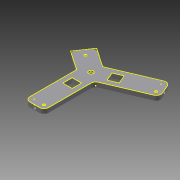
# Autodesk Inventor part: Auto Steering Part
Saved by Autodesk Inventor 2014 (Build 180170000, 170)
## iProperties
Created: 2015-01-15
Part Number: Auto Steering Part
Material: Generic
Document SubType Name: Modeling
Designer: WillHuie
Density: 1 g/cm^3
Appearance: Default
Author: WillHuie
Autodesk Inventor part; units mm, degrees
ref_plane "YZ Plane" through (0, 0, 0) normal (1, 0, 0) x (0, 1, 0)
ref_plane "XZ Plane" through (0, 0, 0) normal (0, 1, 0) x (-1, 0, 0)
ref_plane "XY Plane" through (0, 0, 0) normal (0, 0, 1) x (1, 0, 0)
sketch "Sketch1" plane through (0, 0, 0) normal (0, 1, 0) x (-1, 0, 0)
  line L0 (0, -74.6125) -> (0, -76.2)
  line L1 (0, -76.2) -> (-1.461, -76.8211)
  line L2 (-70.1269, -106.0104) -> (-75.0953, -94.3226)
  line L3 (0, 0) -> (-12.7, 0)
  line L4 (0, 0) -> (12.7, 0)
  line L5 (-75.0953, -94.3226) -> (-12.7, -67.7988)
  line L6 (-12.7, 0) -> (-12.7, -67.7988)
  line L7 (-70.1269, -106.0104) -> (-65.1585, -117.6982)
  line L8 (-65.1585, -117.6982) -> (12.7, -84.6012)
  line L9 (12.7, -84.6012) -> (12.7, 0)
  circle A0 centre (0, -76.2) radius 1.5875
  dimension "d0" = 76.2
  dimension "d1" = 76.2
  dimension "d2" = 113.03
  dimension "d3" = 12.7
  dimension "d4" = 12.7
  dimension "d5" = 12.7
  dimension "d6" = 12.7
  dimension "d7" = 3.175
  constraints: 20 end point, 6 perpendicular, 2 coincident, 2 point on circle, 1 centre point, 1 collinear, 1 parallel, 1 vertical
  measures "d0" distance of L3.start L0.end
  measures "d1" distance of L0.end L2.start
  measures "d2" angle of L0 L1
  measures "d3" distance of L2.start L2.end
  measures "d4" distance of L3.start L3.end
  measures "d5" distance of L3.start L4.end
  measures "d6" distance of L2.start L7.end
  measures "d7" diameter of A0
extrude "Extrusion1" add sketch "Sketch1" along normal blind 6.35
sketch "Sketch2" plane through (-12.7, 0, 0) normal (0, 0, 1) x (1, 0, 0)
  circle A0 centre (12.7, 3.175) radius 1.5875
  point P0 (12.7, 0)
  dimension "d10" = 3.175
  constraints: 1 centre point, 1 coincident
  measures "d10" diameter of A0
extrude "Extrusion2" cut sketch "Sketch2" against normal blind 19.05
sketch "Sketch3" plane through (65.1585, 0, -117.6982) normal (0.9203001, 0, -0.3912131) x (-0.3912131, 0, -0.9203001)
  circle A0 centre (-12.7, 3.175) radius 1.5875
  point P0 (-82.8269, 0)
  dimension "d13" = 3.175
  constraints: 1 centre point, 1 coincident
  measures "d13" diameter of A0
extrude "Extrusion3" cut sketch "Sketch3" against normal blind 19.05
fillet "Fillet1" radius 6.35 1 edges at (-12.7, 3.175, -84.6012)
fillet "Fillet2" radius 6.35 1 edges at (12.7, 3.175, -67.7988)
fillet "Fillet3" radius 6.35 1 edges at (65.1585, 3.175, -117.6982)
fillet "Fillet4" radius 6.35 1 edges at (75.0953, 3.175, -94.3226)
fillet "Fillet5" radius 6.35 1 edges at (12.7, 3.175, 0)
fillet "Fillet6" radius 6.35 1 edges at (-12.7, 3.175, 0)
sketch "Sketch4" plane through (0, 6.35, 0) normal (0, 1, 0) x (1, 0, 0)
  circle A0 centre (0, 76.2) radius 1.5875 projected
  circle A1 centre (0, 76.2) radius 3.175
  point P0 (0, 0)
  dimension "d22" = 6.35
  constraints: 1 centre point, 1 coincident
  measures "d22" diameter of A1
extrude "Extrusion4" cut sketch "Sketch4" against normal blind 1.5875
sketch "Sketch5" plane through (0, 6.35, 0) normal (0, 1, 0) x (1, 0, 0)
  arc A0 (69.2514, 91.8384) -> (72.6111, 100.1665) centre (66.7672, 97.6823) ccw projected
  circle A1 centre (66.7672, 97.6823) radius 1.5875
  point P0 (0, 0)
  dimension "d25" = 3.175
  constraints: 1 centre point, 1 coincident
  measures "d25" diameter of A1
extrude "Extrusion5" cut sketch "Sketch5" against normal blind 6.35
sketch "Sketch6" plane through (0, 0, 0) normal (0, -1, 0) x (1, 0, 0)
  circle A0 centre (66.7672, -97.6823) radius 1.5875 projected
  arc A1 (72.6111, -100.1665) -> (69.2514, -91.8384) centre (66.7672, -97.6823) ccw projected
  circle A2 centre (66.7672, -97.6823) radius 3.175
  point P0 (0, 0)
  dimension "d28" = 6.35
  constraints: 1 centre point, 1 coincident
  measures "d28" diameter of A2
extrude "Extrusion6" cut sketch "Sketch6" against normal blind 1.5875
sketch "Sketch7" plane through (0, 0, 0) normal (0, -1, 0) x (1, 0, 0)
  arc A0 (12.7, -6.35) -> (6.35, 0) centre (6.35, -6.35) ccw projected
  circle A1 centre (6.35, -6.35) radius 1.5875
  point P0 (0, 0)
  dimension "d31" = 3.175
  constraints: 1 centre point, 1 coincident
  measures "d31" diameter of A1
extrude "Extrusion7" cut sketch "Sketch7" against normal blind 6.35
sketch "Sketch8" plane through (0, 0, 0) normal (0, -1, 0) x (1, 0, 0)
  circle A0 centre (6.35, -6.35) radius 1.5875 projected
  arc A1 (12.7, -6.35) -> (6.35, 0) centre (6.35, -6.35) ccw projected
  circle A2 centre (6.35, -6.35) radius 3.175
  point P0 (0, 0)
  dimension "d34" = 6.35
  constraints: 1 centre point, 1 coincident
  measures "d34" diameter of A2
extrude "Extrusion8" cut sketch "Sketch8" against normal blind 1.5875
sketch "Sketch9" plane through (0, 3.175, -19.05) normal (0, 0, 1) x (1, 0, 0)
  circle A0 centre (0, 0) radius 1.5875 projected
  point P0 (0, -3.175)
extrude "Extrusion9" cut sketch "Sketch9" against normal blind 31.75
sketch "Sketch10" plane through (52.5952, 3.175, -98.5578) normal (0.9203001, 0, -0.3912131) x (-0.3912131, 0, -0.9203001)
  circle A0 centre (0, 0) radius 1.5875 projected
  point P0 (-70.1269, -3.175)
extrude "Extrusion10" cut sketch "Sketch10" against normal blind 31.75
sketch "Sketch11" plane through (0, 6.35, 0) normal (0, 1, 0) x (1, 0, 0)
  line L0 (-12.7, 80.4006) -> (-12.7, 6.35) projected
  line L1 (0, 57.15) -> (6.35, 57.15)
  line L2 (6.35, 57.15) -> (6.35, 44.45)
  line L3 (6.35, 44.45) -> (-6.35, 44.45)
  line L4 (-6.35, 44.45) -> (-6.35, 57.15)
  line L5 (-6.35, 57.15) -> (0, 57.15)
  point P0 (0, 0)
  dimension "d41" = 6.35
  dimension "d42" = 12.7
  dimension "d43" = 12.7
  dimension "d44" = 12.7
  constraints: 10 end point, 2 parallel, 2 perpendicular
  measures "d41" distance of L1.start L1.end
  measures "d42" distance of L1.end L2.end
  measures "d43" distance of L2.end L3.end
  measures "d44" distance of L3.end L4.end
extrude "Extrusion11" cut sketch "Sketch11" against normal blind 31.75
sketch "Sketch12" plane through (0, 6.35, 0) normal (0, 1, 0) x (1, 0, 0)
  line L0 (72.6111, 100.1665) -> (67.6427, 111.8543) projected
  line L1 (59.3146, 115.214) -> (-8.8342, 86.2445) projected
  line L2 (29.2195, 88.621) -> (17.5317, 83.6526)
  line L3 (17.5317, 83.6526) -> (15.0475, 89.4965)
  line L4 (15.0475, 89.4965) -> (26.7353, 94.4649)
  line L5 (26.7353, 94.4649) -> (31.7037, 82.7771)
  line L6 (31.7037, 82.7771) -> (20.0159, 77.8087)
  line L7 (20.0159, 77.8087) -> (17.5317, 83.6526)
  point P0 (0, 0)
  point P1 (70.1269, 106.0104)
  dimension "d47" = 57.15
  dimension "d48" = 6.35
  dimension "d49" = 12.7
  dimension "d50" = 12.7
  dimension "d51" = 12.7
  constraints: 12 end point, 3 parallel, 2 midpoint, 2 perpendicular
  measures "d47" distance of point (70.127, 106.01) L2.end
  measures "d48" distance of L2.end L3.end
  measures "d49" distance of L3.end L4.end
  measures "d50" distance of L4.end L5.end
  measures "d51" distance of L5.end L6.end
extrude "Extrusion12" cut sketch "Sketch12" against normal blind 31.75 contours L5 L6 L7 L2
sketch "Sketch13" plane through (0, 6.35, 0) normal (0, 1, 0) x (1, 0, 0)
  line L0 (17.5317, 83.6526) -> (29.2195, 88.621) projected
  line L1 (59.3146, 115.214) -> (-8.8342, 86.2445) projected
  line L2 (17.5317, 83.6526) -> (15.0475, 89.4965)
  line L3 (15.0475, 89.4965) -> (26.7353, 94.4649)
  line L4 (26.7353, 94.4649) -> (29.2195, 88.621)
  point P0 (0, 0)
  dimension "d54" = 6.35
  dimension "d55" = 12.7
  constraints: 6 end point, 2 perpendicular
  measures "d54" distance of L0.start L2.end
  measures "d55" distance of L2.end L3.end
extrude "Extrusion13" cut sketch "Sketch13" against normal blind 31.75
sketch "Sketch14" plane through (6.35, 0, 0) normal (0, 0, 1) x (1, 0, 0)
  circle A0 centre (-6.35, 3.175) radius 1.5875 projected
  circle A1 centre (-6.35, 3.175) radius 2.286
  point P0 (-6.35, 0)
  dimension "d58" = 4.572
  constraints: 1 centre point, 1 coincident
  measures "d58" diameter of A1
extrude "Extrusion14" cut sketch "Sketch14" against normal blind 44.45
sketch "Sketch15" plane through (67.6427, 0, -111.8543) normal (0.9203001, 0, -0.3912131) x (-0.3912131, 0, -0.9203001)
  circle A0 centre (-6.35, 3.175) radius 1.5875 projected
  circle A1 centre (-6.35, 3.175) radius 2.286
  point P0 (-76.4769, 0)
  dimension "d61" = 4.572
  constraints: 1 centre point, 1 coincident
  measures "d61" diameter of A1
extrude "Extrusion15" cut sketch "Sketch15" against normal blind 44.45
sketch "Sketch16" plane through (0, 6.35, 0) normal (0, 1, 0) x (1, 0, 0)
  circle A0 centre (0, 76.2) radius 3.175 projected
  line L0 (59.3146, 115.214) -> (-8.8342, 86.2445) projected
  arc A1 (-8.8342, 86.2445) -> (-12.7, 80.4006) centre (-6.35, 80.4006) ccw projected
  line L1 (-12.7, 80.4006) -> (-12.7, 6.35) projected
  line L2 (-31.4662, 97.6823) -> (-24.3054, 108.171)
  line L3 (-24.3054, 108.171) -> (1.4241, 90.6052)
  line L4 (-31.4662, 97.6823) -> (-38.6269, 87.1936)
  line L5 (-38.6269, 87.1936) -> (-12.7, 69.493)
  line L6 (0, 76.2) -> (-2.6222, 77.9902)
  point P0 (0, 0)
  dimension "d64" = 38.1
  dimension "d65" = 12.7
  dimension "d66" = 12.7
  constraints: 10 end point, 3 perpendicular, 2 point on line, 1 parallel, 2 other
  measures "d64" distance of L6.start L2.start
  measures "d65" distance of L2.start L2.end
  measures "d66" distance of L2.start L4.end
extrude "Extrusion16" add sketch "Sketch16" against normal blind 6.35 contours L0 A1 L1 L5 L4 L2 L3
sketch "Sketch17" plane through (0, 6.35, 0) normal (0, 1, 0) x (1, 0, 0)
  line L0 (-24.3054, 108.171) -> (-38.6269, 87.1936) projected
  line L1 (-38.6269, 87.1936) -> (-12.7, 69.493) projected
  line L2 (-31.4662, 97.6823) -> (-23.5996, 92.3117)
  circle A0 centre (-23.5996, 92.3117) radius 1.5875
  point P0 (0, 0)
  dimension "d69" = 9.525
  dimension "d70" = 3.175
  constraints: 2 end point, 1 centre point, 1 coincident, 1 midpoint, 1 parallel
  measures "d69" distance of L2.start L2.end
  measures "d70" diameter of A0
extrude "Extrusion17" cut sketch "Sketch17" against normal blind 6.35
sketch "Sketch18" plane through (0, 6.35, 0) normal (0, 1, 0) x (1, 0, 0)
  circle A0 centre (-23.5996, 92.3117) radius 1.5875 projected
  line L0 (26.7353, 94.4649) -> (31.7037, 82.7771) projected
  line L1 (31.7037, 82.7771) -> (20.0159, 77.8087) projected
  line L2 (20.0159, 77.8087) -> (15.0475, 89.4965) projected
  line L3 (15.0475, 89.4965) -> (26.7353, 94.4649) projected
  line L4 (-6.35, 44.45) -> (-6.35, 57.15) projected
  line L5 (-6.35, 57.15) -> (6.35, 57.15) projected
  line L6 (6.35, 57.15) -> (6.35, 44.45) projected
  line L7 (6.35, 44.45) -> (-6.35, 44.45) projected
  circle A1 centre (6.35, 6.35) radius 1.5875 projected
  circle A2 centre (66.7672, 97.6823) radius 1.5875 projected
  circle A3 centre (0, 76.2) radius 3.175 projected
  arc A4 (-12.7, 6.35) -> (-6.35, 0) centre (-6.35, 6.35) ccw projected
  line L8 (-6.35, 0) -> (6.35, 0) projected
  arc A5 (6.35, 0) -> (12.7, 6.35) centre (6.35, 6.35) ccw projected
  line L9 (12.7, 6.35) -> (12.7, 63.5983) projected
  arc A6 (16.5658, 69.4422) -> (12.7, 63.5983) centre (19.05, 63.5983) ccw projected
  line L10 (16.5658, 69.4422) -> (69.2514, 91.8384) projected
  arc A7 (69.2514, 91.8384) -> (72.6111, 100.1665) centre (66.7672, 97.6823) ccw projected
  line L11 (72.6111, 100.1665) -> (67.6427, 111.8543) projected
  arc A8 (67.6427, 111.8543) -> (59.3146, 115.214) centre (61.7988, 109.3701) ccw projected
  line L12 (59.3146, 115.214) -> (1.4241, 90.6052) projected
  line L13 (1.4241, 90.6052) -> (-24.3054, 108.171) projected
  line L14 (-24.3054, 108.171) -> (-38.6269, 87.1936) projected
  line L15 (-38.6269, 87.1936) -> (-12.7, 69.493) projected
  line L16 (-12.7, 69.493) -> (-12.7, 6.35) projected
  point P0 (0, 0)
sketch "Sketch19" plane through (0, 0, 0) normal (0, -1, 0) x (1, 0, 0)
  circle A0 centre (-23.5996, -92.3117) radius 1.5875 projected
  circle A1 centre (-23.5996, -92.3117) radius 3.175
  point P0 (0, 0)
  dimension "d73" = 6.35
  constraints: 1 centre point, 1 coincident
  measures "d73" diameter of A1
extrude "Extrusion18" cut sketch "Sketch19" against normal blind 1.5875
fillet "Fillet7" radius 6.35 1 edges at (-24.3054, 3.175, -108.171)
fillet "Fillet8" radius 6.35 1 edges at (-38.6269, 3.175, -87.1936)
fillet "Fillet9" radius 6.35 1 edges at (1.4241, 3.175, -90.6052)
fillet "Fillet10" radius 6.35 1 edges at (-12.7, 3.175, -69.493)
body "Solid1"
